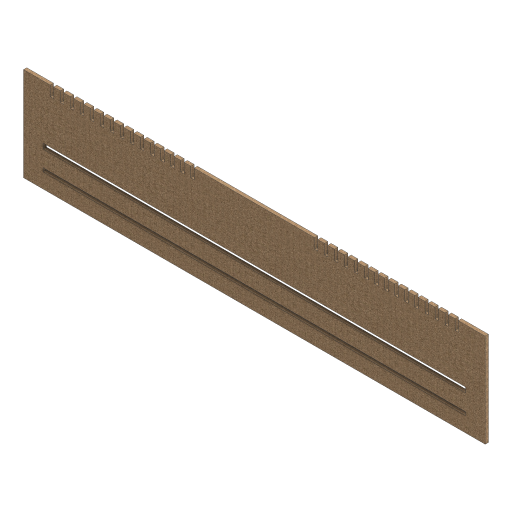
# Autodesk Inventor part: PARED_MODULAR
Saved by Autodesk Inventor 2024.2 (Build 282272000, 272)
## iProperties
Created: 2024-07-19
Part Number: PARED_MODULAR
Material: MDF Medium Density Fiberboard
Document SubType Name: Modeling
Designer: jrcer
Density: 0.8 g/cm^3
Appearance: Cardboard - Corrugated
Author: jrcer
Autodesk Inventor part; units mm, degrees
ref_plane "YZ Plane" through (0, 0, 0) normal (1, 0, 0) x (0, 1, 0)
ref_plane "XZ Plane" through (0, 0, 0) normal (0, 1, 0) x (-1, 0, 0)
ref_plane "XY Plane" through (0, 0, 0) normal (0, 0, 1) x (1, 0, 0)
sketch "Sketch1" plane through (0, 0, 0) normal (0, 0, 1) x (1, 0, 0)
  line L0 (0, 0) -> (460, 0)
  line L1 (460, 0) -> (460, 93.35)
  line L2 (460, 93.35) -> (0, 93.35)
  line L3 (0, 93.35) -> (0, 0)
  line L4 (19.5, 18.35) -> (440.5, 18.35)
  line L5 (440.5, 18.35) -> (440.5, 15)
  line L6 (440.5, 15) -> (19.5, 15)
  line L7 (19.5, 15) -> (19.5, 18.35)
  line L8 (26.8, 93.35) -> (30, 93.35)
  line L9 (30, 93.35) -> (30, 83.35)
  line L10 (30, 83.35) -> (26.8, 83.35)
  line L11 (26.8, 83.35) -> (26.8, 93.35)
  line L12 (230, 0) -> (230, 93.35) construction
  line L13 (40, 93.35) -> (40, 83.35)
  line L14 (40, 83.35) -> (36.8, 83.35)
  line L15 (36.8, 83.35) -> (36.8, 93.35)
  line L16 (36.8, 93.35) -> (40, 93.35)
  line L17 (50, 93.35) -> (50, 83.35)
  line L18 (50, 83.35) -> (46.8, 83.35)
  line L19 (46.8, 83.35) -> (46.8, 93.35)
  line L20 (46.8, 93.35) -> (50, 93.35)
  line L21 (60, 93.35) -> (60, 83.35)
  line L22 (60, 83.35) -> (56.8, 83.35)
  line L23 (56.8, 83.35) -> (56.8, 93.35)
  line L24 (56.8, 93.35) -> (60, 93.35)
  line L25 (70, 93.35) -> (70, 83.35)
  line L26 (70, 83.35) -> (66.8, 83.35)
  line L27 (66.8, 83.35) -> (66.8, 93.35)
  line L28 (66.8, 93.35) -> (70, 93.35)
  line L29 (80, 93.35) -> (80, 83.35)
  line L30 (80, 83.35) -> (76.8, 83.35)
  line L31 (76.8, 83.35) -> (76.8, 93.35)
  line L32 (76.8, 93.35) -> (80, 93.35)
  line L33 (90, 93.35) -> (90, 83.35)
  line L34 (90, 83.35) -> (86.8, 83.35)
  line L35 (86.8, 83.35) -> (86.8, 93.35)
  line L36 (86.8, 93.35) -> (90, 93.35)
  line L37 (100, 93.35) -> (100, 83.35)
  line L38 (100, 83.35) -> (96.8, 83.35)
  line L39 (96.8, 83.35) -> (96.8, 93.35)
  line L40 (96.8, 93.35) -> (100, 93.35)
  line L41 (110, 93.35) -> (110, 83.35)
  line L42 (110, 83.35) -> (106.8, 83.35)
  line L43 (106.8, 83.35) -> (106.8, 93.35)
  line L44 (106.8, 93.35) -> (110, 93.35)
  line L45 (120, 93.35) -> (120, 83.35)
  line L46 (120, 83.35) -> (116.8, 83.35)
  line L47 (116.8, 83.35) -> (116.8, 93.35)
  line L48 (116.8, 93.35) -> (120, 93.35)
  line L49 (130, 93.35) -> (130, 83.35)
  line L50 (130, 83.35) -> (126.8, 83.35)
  line L51 (126.8, 83.35) -> (126.8, 93.35)
  line L52 (126.8, 93.35) -> (130, 93.35)
  line L53 (140, 93.35) -> (140, 83.35)
  line L54 (140, 83.35) -> (136.8, 83.35)
  line L55 (136.8, 83.35) -> (136.8, 93.35)
  line L56 (136.8, 93.35) -> (140, 93.35)
  line L57 (150, 93.35) -> (150, 83.35)
  line L58 (150, 83.35) -> (146.8, 83.35)
  line L59 (146.8, 83.35) -> (146.8, 93.35)
  line L60 (146.8, 93.35) -> (150, 93.35)
  line L61 (160, 93.35) -> (160, 83.35)
  line L62 (160, 83.35) -> (156.8, 83.35)
  line L63 (156.8, 83.35) -> (156.8, 93.35)
  line L64 (156.8, 93.35) -> (160, 93.35)
  line L65 (170, 93.35) -> (170, 83.35)
  line L66 (170, 83.35) -> (166.8, 83.35)
  line L67 (166.8, 83.35) -> (166.8, 93.35)
  line L68 (166.8, 93.35) -> (170, 93.35)
  line L69 (433.2, 93.35) -> (430, 93.35)
  line L70 (430, 93.35) -> (430, 83.35)
  line L71 (430, 83.35) -> (433.2, 83.35)
  line L72 (433.2, 83.35) -> (433.2, 93.35)
  line L73 (420, 93.35) -> (420, 83.35)
  line L74 (420, 83.35) -> (423.2, 83.35)
  line L75 (423.2, 83.35) -> (423.2, 93.35)
  line L76 (423.2, 93.35) -> (420, 93.35)
  line L77 (410, 93.35) -> (410, 83.35)
  line L78 (410, 83.35) -> (413.2, 83.35)
  line L79 (413.2, 83.35) -> (413.2, 93.35)
  line L80 (413.2, 93.35) -> (410, 93.35)
  line L81 (400, 93.35) -> (400, 83.35)
  line L82 (400, 83.35) -> (403.2, 83.35)
  line L83 (403.2, 83.35) -> (403.2, 93.35)
  line L84 (403.2, 93.35) -> (400, 93.35)
  line L85 (390, 93.35) -> (390, 83.35)
  line L86 (390, 83.35) -> (393.2, 83.35)
  line L87 (393.2, 83.35) -> (393.2, 93.35)
  line L88 (393.2, 93.35) -> (390, 93.35)
  line L89 (380, 93.35) -> (380, 83.35)
  line L90 (380, 83.35) -> (383.2, 83.35)
  line L91 (383.2, 83.35) -> (383.2, 93.35)
  line L92 (383.2, 93.35) -> (380, 93.35)
  line L93 (370, 93.35) -> (370, 83.35)
  line L94 (370, 83.35) -> (373.2, 83.35)
  line L95 (373.2, 83.35) -> (373.2, 93.35)
  line L96 (373.2, 93.35) -> (370, 93.35)
  line L97 (360, 93.35) -> (360, 83.35)
  line L98 (360, 83.35) -> (363.2, 83.35)
  line L99 (363.2, 83.35) -> (363.2, 93.35)
  line L100 (363.2, 93.35) -> (360, 93.35)
  line L101 (350, 93.35) -> (350, 83.35)
  line L102 (350, 83.35) -> (353.2, 83.35)
  line L103 (353.2, 83.35) -> (353.2, 93.35)
  line L104 (353.2, 93.35) -> (350, 93.35)
  line L105 (340, 93.35) -> (340, 83.35)
  line L106 (340, 83.35) -> (343.2, 83.35)
  line L107 (343.2, 83.35) -> (343.2, 93.35)
  line L108 (343.2, 93.35) -> (340, 93.35)
  line L109 (330, 93.35) -> (330, 83.35)
  line L110 (330, 83.35) -> (333.2, 83.35)
  line L111 (333.2, 83.35) -> (333.2, 93.35)
  line L112 (333.2, 93.35) -> (330, 93.35)
  line L113 (320, 93.35) -> (320, 83.35)
  line L114 (320, 83.35) -> (323.2, 83.35)
  line L115 (323.2, 83.35) -> (323.2, 93.35)
  line L116 (323.2, 93.35) -> (320, 93.35)
  line L117 (310, 93.35) -> (310, 83.35)
  line L118 (310, 83.35) -> (313.2, 83.35)
  line L119 (313.2, 83.35) -> (313.2, 93.35)
  line L120 (313.2, 93.35) -> (310, 93.35)
  line L121 (300, 93.35) -> (300, 83.35)
  line L122 (300, 83.35) -> (303.2, 83.35)
  line L123 (303.2, 83.35) -> (303.2, 93.35)
  line L124 (303.2, 93.35) -> (300, 93.35)
  line L125 (290, 93.35) -> (290, 83.35)
  line L126 (290, 83.35) -> (293.2, 83.35)
  line L127 (293.2, 83.35) -> (293.2, 93.35)
  line L128 (293.2, 93.35) -> (290, 93.35)
  line L129 (19.5, 39.6635) -> (440.5, 39.6635)
  line L130 (440.5, 39.6635) -> (440.5, 34.6635)
  line L131 (440.5, 34.6635) -> (19.5, 34.6635)
  line L132 (19.5, 34.6635) -> (19.5, 39.6635)
  point P0 (230, 15)
  point P1 (170, 93.35)
  point P2 (166.8, 93.35)
  point P3 (160, 93.35)
  point P4 (156.8, 93.35)
  point P5 (150, 93.35)
  point P6 (146.8, 93.35)
  point P7 (140, 93.35)
  point P8 (136.8, 93.35)
  point P9 (130, 93.35)
  point P10 (126.8, 93.35)
  point P11 (120, 93.35)
  point P12 (116.8, 93.35)
  point P13 (110, 93.35)
  point P14 (106.8, 93.35)
  point P15 (100, 93.35)
  point P16 (96.8, 93.35)
  point P17 (90, 93.35)
  point P18 (86.8, 93.35)
  point P19 (80, 93.35)
  point P20 (76.8, 93.35)
  point P21 (70, 93.35)
  point P22 (66.8, 93.35)
  point P23 (60, 93.35)
  point P24 (56.8, 93.35)
  point P25 (50, 93.35)
  point P26 (46.8, 93.35)
  point P27 (40, 93.35)
  point P28 (36.8, 93.35)
  point P29 (30, 93.35)
  point P30 (230, 39.6635)
  dimension "d0" = 460
  dimension "d2" = 421
  dimension "d3" = 3.35
  dimension "d4" = 75
  dimension "d5" = 15
  dimension "d6" = 3.2
  dimension "d7" = 10
  dimension "d8" = 26.8
  dimension "d11" = 10
  dimension "d18" = 5
  dimension "d19" = 16.3135
  constraints: 264 end point, 60 symmetric about line, 56 horizontal alignment, 36 parallel, 28 collinear, 5 horizontal, 4 perpendicular, 3 midpoint, 2 vertical alignment, 1 vertical, 5 other
  measures "d0" distance of L3.start L1.end
  measures "d2" distance of L5.end L6.end
  measures "d3" distance between parallel lines of L6 L4
  measures "d5" distance between parallel lines of L0 L6
  measures "d6" distance of L9.end L10.end
  measures "d7" distance of L8.end L9.end
  measures "d8" distance between parallel lines of L3 L11
  measures "d11" distance of L9.end L13.end
  measures "d18" distance between parallel lines of L131 L129
  measures "d19" distance between parallel lines of L4 L131
extrude "Extrusion1" add sketch "Sketch1" along normal blind 3.2 contours L3 L2 L11 L10 L9 L15 L14 L13 L19 L18 L17 L23 L22 L21 L27 L26 L25 L31 L30 L29 L35 L34 L33 L39 L38 L37 L43 L42 L41 L47 L46 L45 L51 L50 L49 L55 L54 L53 L59 L58 L57 L63 L62 L61 L67 L66 L65 L125 L126 L127 L121 L122 L123 L117 L118 L119 L113 L114 L115 L109 L110 L111 L105 L106 L107 L101 L102 L103 L97 L98 L99 L93 L94 L95 L89 L90 L91 L85 L86 L87 L81 L82 L83 L77 L78 L79 L73 L74 L75 L70 L71 L72 L1 L0
body "Solid1"
